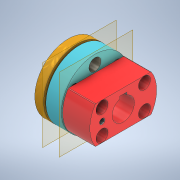
# Autodesk Inventor part: Муфта_Корпус
Saved by Autodesk Inventor 2021 (Build 250183000, 183)
## iProperties
Created: 2023-04-14
Part Number: Муфта_Корпус
Material: Сталь, углеродистая
Document SubType Name: Modeling
Designer: gdevc
Density: 7.85 g/cm^3
Appearance: С умеренной полировкой
Author: gdevc
Autodesk Inventor part; units mm, degrees
ref_plane "YZ Plane" through (0, 0, 0) normal (1, 0, 0) x (0, 1, 0)
ref_plane "XZ Plane" through (0, 0, 0) normal (0, 1, 0) x (-1, 0, 0)
ref_plane "XY Plane" through (0, 0, 0) normal (0, 0, 1) x (1, 0, 0)
sketch "Эскиз1" plane through (0, 0, 0) normal (0, 0, 1) x (1, 0, 0)
  line L0 (0, 25) -> (40.6981, 25)
  line L1 (0, 0) -> (36.5301, 0)
  line L2 (0, 25) -> (0, 37.5)
  line L3 (0, 37.5) -> (25.6981, 37.5)
  line L4 (25.6981, 37.5) -> (25.6981, 75)
  line L5 (25.6981, 75) -> (38.5952, 75)
  line L6 (38.5952, 75) -> (45.6981, 75)
  line L7 (45.6981, 75) -> (45.6981, 30)
  line L8 (45.6981, 30) -> (40.6981, 30)
  line L9 (40.6981, 30) -> (40.6981, 25)
  point P0 (25.6981, 56.25)
  dimension "d1" = 50
  dimension "d2" = 75
  dimension "d3" = 5
  dimension "d4" = 5
  dimension "d5" = 20
  dimension "d6" = 150
  constraints: 20 end point, 6 perpendicular, 3 horizontal, 1 midpoint, 1 point on line, 1 vertical
  measures "d1" diameter of L0 L1
  measures "d2" diameter of L3 L1
  measures "d3" distance between parallel lines of L7 L9
  measures "d4" distance between parallel lines of L0 L8
  measures "d5" distance between parallel lines of L7 L4
  measures "d6" diameter of L5 L1
revolve "Вращение1" add sketch "Эскиз1" angle 360 about axis through (0, 0, 0) along (1, 0, 0)
ref_plane "РабПлоскость1" through (50.6981, 0, 0) normal (1, 0, 0) x (0, 0, -1)
sketch "Эскиз2" plane through (0, 0, 0) normal (0, 0, 1) x (1, 0, 0)
  line L0 (55.6981, 30) -> (85.6981, 30)
  line L1 (85.6981, 30) -> (85.6981, 75)
  line L2 (85.6981, 75) -> (50.6981, 75)
  line L3 (50.6981, 75) -> (50.6981, 35)
  line L4 (0, 0) -> (146.6296, 0)
  line L5 (50.6981, 105) -> (50.6981, -105) projected
  line L6 (50.6981, 55) -> (85.6981, 55)
  line L7 (50.6981, 35) -> (50.6981, 30)
  line L8 (55.6981, 30) -> (50.6981, 30)
  point P0 (50.6981, 0)
  dimension "d10" = 60
  dimension "d11" = 150
  dimension "d14" = 35
  constraints: 16 end point, 5 perpendicular, 4 point on line, 2 midpoint, 1 horizontal
  measures "d10" diameter of L0 L4
  measures "d11" diameter of L2 L4
  measures "d14" distance between parallel lines of L3 L1
revolve "Вращение2" add sketch "Эскиз2" angle 360 about axis through (0, 0, 0) along (1, 0, 0)
ref_plane "РабПлоскость2" through (88.1981, 0, 0) normal (1, 0, 0) x (0, 0, -1)
sketch "Эскиз3" plane through (0, 0, 0) normal (0, 0, 1) x (1, 0, 0)
  line L0 (88.1981, 105) -> (88.1981, -105) projected
  line L1 (88.1981, 25) -> (149.1981, 25)
  line L2 (149.1981, 25) -> (149.1981, 75)
  line L3 (149.1981, 75) -> (88.1981, 75)
  line L4 (88.1981, 25) -> (88.1981, 75)
  line L5 (88.1981, 0) -> (129.5477, 0)
  point P0 (0, 0)
  dimension "d17" = 50
  dimension "d18" = 150
  dimension "d19" = 61
  constraints: 10 end point, 2 horizontal, 2 perpendicular, 2 point on line, 1 collinear, 1 midpoint
  measures "d17" diameter of L1 L5
  measures "d18" diameter of L3 L5
  measures "d19" distance of L2.end L3.end
revolve "Вращение3" add sketch "Эскиз3" angle 360 about axis through (88.1981, 0, 0) along (1, 0, 0)
sketch "Эскиз4" plane through (149.1981, 0, 0) normal (1, 0, 0) x (0, 0, -1)
  circle A0 centre (0, 0) radius 55
  circle A1 centre (0, 0) radius 75 projected
  circle A2 centre (0, 55) radius 13.5
  circle A3 centre (47.6314, 27.5) radius 13.5
  circle A4 centre (0, 0) radius 55
  circle A5 centre (47.6314, -27.5) radius 13.5
  circle A6 centre (0, 0) radius 55
  circle A7 centre (0, -55) radius 13.5
  circle A8 centre (0, 0) radius 55
  circle A9 centre (-47.6314, -27.5) radius 13.5
  circle A10 centre (0, 0) radius 55
  circle A11 centre (-47.6314, 27.5) radius 13.5
  circle A12 centre (0, 0) radius 55
  dimension "d21" = 110
  dimension "d23" = 27
  dimension "d24" = 55
  dimension "d27" = 360
  constraints: 6 centre point, 3 coincident, 2 vertical alignment, 39 other
  measures "d23" diameter of A2
  measures "d24" distance of point (0, 0) A2.centre
extrude "Выдавливание1" cut sketch "Эскиз4" against normal up to surface (98.5 mm away) contours A3 A0 | A0 A3 | A5 A0 | A0 A5 | A2 A0 | A0 A2 | A7 A0 | A0 A7 | A11 A0 | A0 A11 | A9 A0 | A0 A9
sketch "Эскиз6" plane through (0, 0, 0) normal (0, 0, 1) x (1, 0, 0)
  line L0 (85.6981, 68.5) -> (85.6981, 41.5) projected
  line L1 (50.6981, 41.5) -> (50.6981, 68.5) projected
  line L2 (85.6981, 68.5) -> (50.6981, 68.5) projected
  line L3 (85.6981, 41.5) -> (50.6981, 41.5) projected
  line L4 (50.6981, 41.5) -> (50.6981, 68.5) projected
  line L5 (50.6981, 55) -> (18.7693, 55)
  line L6 (25.6981, -75) -> (25.6981, 75) projected
  line L7 (25.6981, 55) -> (25.6981, 61)
  line L8 (25.6981, 61) -> (45.6981, 62)
  line L9 (45.6981, -75) -> (45.6981, 75) projected
  line L10 (45.6981, 55) -> (45.6981, 62)
  point P0 (0, 0)
  dimension "d38" = 6
  dimension "d39" = 7
  dimension "d44" = 27
  constraints: 8 end point, 5 point on line, 1 horizontal, 1 midpoint, 1 parallel
  measures "d38" distance of L7.end L7.start
  measures "d39" distance of L10.start L8.end
  measures "d44" diameter of L3 L5
revolve "Вращение4" cut sketch "Эскиз6" angle 360 about axis through (50.6981, 55, 0) along (-1, 0, 0) contours L5 L6 L8 L9
sketch "Эскиз7" plane through (25.6981, 0, 0) normal (-1, 0, 0) x (0, 0, 1)
  circle A0 centre (0, 55) radius 7 projected
  circle A1 centre (0, 0) radius 55
  constraints: 1 coincident, 1 vertical alignment, 2 other
pattern_circular "Круговой массив1" count 6 over 360 about axis through (20.349, 0, 0) along (1, 0, 0) of "Вращение4"
sketch "Эскиз8" plane through (149.1981, 0, 0) normal (1, 0, 0) x (0, 0, -1)
  circle A0 centre (0, 0) radius 75 projected
  line L0 (-62.472, 41.5) -> (62.472, 41.5)
  line L1 (62.472, 41.5) -> (62.472, -41.5)
  line L2 (62.472, -41.5) -> (-62.472, -41.5)
  line L3 (-62.472, -41.5) -> (-62.472, 41.5)
  circle A1 centre (0, 55) radius 13.5 projected
  circle A2 centre (0, -55) radius 13.5 projected
  point P0 (0, -41.5)
  point P1 (0, 41.5)
  point P2 (62.472, 41.5)
  constraints: 8 end point, 2 parallel, 2 point on circle, 2 tangent, 1 horizontal, 1 perpendicular
extrude "Выдавливание3" cut sketch "Эскиз8" against normal up to surface (61 mm away) contours L0 A0 | A0 L2
fillet "Сопряжение1" radius 2 4 edges at (118.6981, 41.5, -62.472) (118.6981, 41.5, 62.472) (118.6981, -41.5, 62.472) (118.6981, -41.5, -62.472)
sketch "Эскиз9" plane through (149.1981, 0, 0) normal (1, 0, 0) x (0, 0, -1)
  circle A0 centre (0, 0) radius 25 projected
  circle A1 centre (0, 0) radius 25 projected
  circle A2 centre (0, 0) radius 47.3
  circle A3 centre (-47.3, 0) radius 5
  dimension "d48" = 94.6
  dimension "d49" = 10
  constraints: 1 centre point, 1 coincident, 1 horizontal alignment, 2 other
  measures "d49" diameter of A3
extrude "Выдавливание4" cut sketch "Эскиз9" against normal blind 70 contours A3 A2 | A2 A3 picked at (-45.6137, 0) picked at (-48.9341, -0.2076)
thread "Резьба1" size "M10x1.5" class "6H" standard "ISO Metric profile" length 18
chamfer "Фаска2" distance 1 angle 45 1 edges at (149.1981, 0, 52.3)
sketch "Эскиз10" plane through (149.1981, 0, 0) normal (1, 0, 0) x (0, 0, -1)
  circle A0 centre (0, 0) radius 25 projected
  line L0 (-8, 29.2) -> (8, 29.2)
  line L1 (8, 29.2) -> (8, 14.745)
  line L2 (8, 14.745) -> (-8, 14.745)
  line L3 (-8, 14.745) -> (-8, 29.2)
  circle A1 centre (0, 0) radius 25 projected
  line L4 (0, 25) -> (-8, 25) construction
  dimension "d63" = 16
  dimension "d64" = 8
  dimension "d65" = 4.2
  constraints: 10 end point, 2 horizontal, 2 parallel, 2 perpendicular, 1 point on line, 1 tangent, 1 vertical alignment, 1 other
  measures "d63" distance between parallel lines of L1 L3
  measures "d64" distance from line of point (0, 0) L3
  measures "d65" distance between parallel lines of L4 L0
extrude "Выдавливание5" cut sketch "Эскиз10" against normal up to surface (63.5 mm away) contours L1 L2 L3 A0 | A0 L3 L0 L1 picked at (0.903, 18.1143)
equation "\"d2\" = 1.5 * d1"
equation "\"d64\" = 0.5 * d63"
